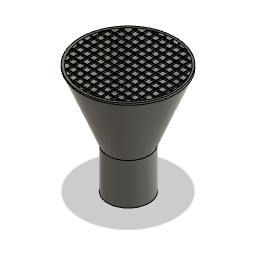
nose1 (Autodesk Fusion 360 design; units mm, degrees)
Autodesk Fusion 360 part; units mm, degrees
(part 1 of 3)
sketch "Sketch1" plane through (0, 0, 0) normal (0, 1, 0) x (1, 0, 0)
  circle A0 centre (0, 0) radius 15
  dimension "d1" = 30
  constraint coincident A0.centre origin
  measures "d1" diameter of A0
extrude "Extrude1" add sketch "Sketch1" along normal blind 30
ref_plane "WorkPlane1" through (0, 80, 0) normal (0, 1, 0) x (1, 0, 0)
sketch "Sketch2" plane through (0, 80, 0) normal (0, 1, 0) x (1, 0, 0)
  circle A0 centre (0, 0) radius 35
  constraint coincident A0.centre origin
loft "Loft1" add profiles "Sketch2" section 1 face at (0.9463, 30, 5.6032) section 2
shell "Shell1" thickness 2 removed faces 1 at (8.8451, 80, 11.8425)
sketch "Sketch3" plane through (0, 0, 0) normal (0, -1, 0) x (1, 0, 0)
  circle A0 centre (0, 0) radius 15
  circle A1 centre (0, 0) radius 13.5
  line L0 (-0.3, -13) -> (0.3, -13)
  line L1 (0.3, -13) -> (0.3, -16.7383)
  line L2 (0.3, -16.7383) -> (-0.3, -16.7383)
  line L3 (-0.3, -16.7383) -> (-0.3, -13)
  dimension "d6" = 27
  constraint coincident A0.centre A1.centre
  constraint horizontal L0
  constraint vertical L1
  constraint horizontal L2
  constraint vertical L3
  measures "d6" diameter of A1
extrude "Extrude2" cut sketch "Sketch3" against normal blind 37 contours A0 A1 L1 L3 | A0 L1 L2 L3 | A1 L0 L1 L3 | A1 L0 L1 L3 picked at (0.2333, -13.9978)
ref_plane "WorkPlane2" through (0, 81, 0) normal (0, 1, 0) x (0, 0, 1)
sketch "Sketch4" plane through (0, 81, 0) normal (0, 1, 0) x (1, 0, 0)
  circle A0 centre (0, 0) radius 35 construction
  line L0 (5, -30) -> (0.5, -30)
  line L1 (0.5, -30) -> (0.5, -25.5)
  line L2 (0.5, -25.5) -> (5, -25.5)
  line L3 (5, -25.5) -> (5, -30)
  line L4 (-4.5, -30) -> (-4.5, -25.5)
  line L5 (0, -25.5) -> (0, -30)
  line L6 (0, -30) -> (-4.5, -30)
  line L7 (-4.5, -25.5) -> (0, -25.5)
  line L8 (-14.5, -30) -> (-14.5, -25.5)
  line L9 (-9.5, -25.5) -> (-5, -25.5)
  line L10 (-10, -25.5) -> (-10, -30)
  line L11 (-14.5, -25.5) -> (-10, -25.5)
  line L12 (-5, -30) -> (-9.5, -30)
  line L13 (-5, -25.5) -> (-5, -30)
  line L14 (-9.5, -30) -> (-9.5, -25.5)
  line L15 (-10, -30) -> (-14.5, -30)
  line L16 (-24.5, -30) -> (-24.5, -25.5)
  line L17 (-19.5, -25.5) -> (-15, -25.5)
  line L18 (-20, -25.5) -> (-20, -30)
  line L19 (-24.5, -25.5) -> (-20, -25.5)
  line L20 (-15, -30) -> (-19.5, -30)
  line L21 (-15, -25.5) -> (-15, -30)
  line L22 (-19.5, -30) -> (-19.5, -25.5)
  line L23 (-20, -30) -> (-24.5, -30)
  line L24 (-34.5, -30) -> (-34.5, -25.5)
  line L25 (-29.5, -25.5) -> (-25, -25.5)
  line L26 (-30, -25.5) -> (-30, -30)
  line L27 (-34.5, -25.5) -> (-30, -25.5)
  line L28 (-25, -30) -> (-29.5, -30)
  line L29 (-25, -25.5) -> (-25, -30)
  line L30 (-29.5, -30) -> (-29.5, -25.5)
  line L31 (-30, -30) -> (-34.5, -30)
  line L32 (5.5, -30) -> (5.5, -25.5)
  line L33 (10.5, -25.5) -> (15, -25.5)
  line L34 (10, -25.5) -> (10, -30)
  line L35 (5.5, -25.5) -> (10, -25.5)
  line L36 (15, -30) -> (10.5, -30)
  line L37 (15, -25.5) -> (15, -30)
  line L38 (10.5, -30) -> (10.5, -25.5)
  line L39 (10, -30) -> (5.5, -30)
  line L40 (15.5, -30) -> (15.5, -25.5)
  line L41 (20.5, -25.5) -> (25, -25.5)
  line L42 (20, -25.5) -> (20, -30)
  line L43 (15.5, -25.5) -> (20, -25.5)
  line L44 (25, -30) -> (20.5, -30)
  line L45 (25, -25.5) -> (25, -30)
  line L46 (20.5, -30) -> (20.5, -25.5)
  line L47 (20, -30) -> (15.5, -30)
  line L48 (25.5, -30) -> (25.5, -25.5)
  line L49 (30.5, -25.5) -> (35, -25.5)
  line L50 (30, -25.5) -> (30, -30)
  line L51 (25.5, -25.5) -> (30, -25.5)
  line L52 (35, -30) -> (30.5, -30)
  line L53 (35, -25.5) -> (35, -30)
  line L54 (30.5, -30) -> (30.5, -25.5)
  line L55 (30, -30) -> (25.5, -30)
  line L56 (35, -25) -> (30.5, -25)
  line L57 (25, -20.5) -> (25, -25)
  line L58 (-14.5, -25) -> (-14.5, -20.5)
  line L59 (0.5, -25) -> (0.5, -20.5)
  line L60 (10.5, -20.5) -> (15, -20.5)
  line L61 (30.5, -25) -> (30.5, -20.5)
  line L62 (25.5, -20.5) -> (30, -20.5)
  line L63 (35, -20.5) -> (35, -25)
  line L64 (-5, -20.5) -> (-5, -25)
  line L65 (0, -25) -> (-4.5, -25)
  line L66 (5.5, -25) -> (5.5, -20.5)
  line L67 (15, -20.5) -> (15, -25)
  line L68 (30.5, -20.5) -> (35, -20.5)
  line L69 (20, -25) -> (15.5, -25)
  line L70 (20, -20.5) -> (20, -25)
  line L71 (5.5, -20.5) -> (10, -20.5)
  line L72 (10.5, -25) -> (10.5, -20.5)
  line L73 (10, -20.5) -> (10, -25)
  line L74 (0.5, -20.5) -> (5, -20.5)
  line L75 (-15, -20.5) -> (-15, -25)
  line L76 (-19.5, -20.5) -> (-15, -20.5)
  line L77 (-24.5, -25) -> (-24.5, -20.5)
  line L78 (-4.5, -25) -> (-4.5, -20.5)
  line L79 (-29.5, -25) -> (-29.5, -20.5)
  line L80 (-9.5, -20.5) -> (-5, -20.5)
  line L81 (-34.5, -25) -> (-34.5, -20.5)
  line L82 (-25, -20.5) -> (-25, -25)
  line L83 (-34.5, -20.5) -> (-30, -20.5)
  line L84 (-20, -25) -> (-24.5, -25)
  line L85 (20.5, -20.5) -> (25, -20.5)
  line L86 (5, -25) -> (0.5, -25)
  line L87 (-15, -25) -> (-19.5, -25)
  line L88 (-9.5, -25) -> (-9.5, -20.5)
  line L89 (30, -25) -> (25.5, -25)
  line L90 (25.5, -25) -> (25.5, -20.5)
  line L91 (30, -20.5) -> (30, -25)
  line L92 (-10, -20.5) -> (-10, -25)
  line L93 (10, -25) -> (5.5, -25)
  line L94 (-5, -25) -> (-9.5, -25)
  line L95 (15.5, -20.5) -> (20, -20.5)
  line L96 (-30, -25) -> (-34.5, -25)
  line L97 (15, -25) -> (10.5, -25)
  line L98 (-14.5, -20.5) -> (-10, -20.5)
  line L99 (-10, -25) -> (-14.5, -25)
  line L100 (20.5, -25) -> (20.5, -20.5)
  line L101 (25, -25) -> (20.5, -25)
  line L102 (15.5, -25) -> (15.5, -20.5)
  line L103 (5, -20.5) -> (5, -25)
  line L104 (-24.5, -20.5) -> (-20, -20.5)
  line L105 (-20, -20.5) -> (-20, -25)
  line L106 (-29.5, -20.5) -> (-25, -20.5)
  line L107 (-30, -20.5) -> (-30, -25)
  line L108 (-19.5, -25) -> (-19.5, -20.5)
  line L109 (0, -20.5) -> (0, -25)
  line L110 (-4.5, -20.5) -> (0, -20.5)
  line L111 (-25, -25) -> (-29.5, -25)
  line L112 (-5, -15) -> (-9.5, -15)
  line L113 (0, -10.5) -> (0, -15)
  line L114 (5, -15) -> (0.5, -15)
  line L115 (-9.5, -10.5) -> (-5, -10.5)
  line L116 (0.5, -15) -> (0.5, -10.5)
  line L117 (10, -15) -> (5.5, -15)
  line L118 (-4.5, -15) -> (-4.5, -10.5)
  line L119 (-10, -10.5) -> (-10, -15)
  line L120 (0, -15) -> (-4.5, -15)
  line L121 (-9.5, -15) -> (-9.5, -10.5)
  line L122 (15, -15) -> (10.5, -15)
  line L123 (15.5, -15) -> (15.5, -10.5)
  line L124 (30, -15.5) -> (30, -20)
  line L125 (-19.5, -20) -> (-19.5, -15.5)
  line L126 (20, -15) -> (15.5, -15)
  line L127 (10.5, -10.5) -> (15, -10.5)
  line L128 (-34.5, -15.5) -> (-30, -15.5)
  line L129 (-25, -15) -> (-29.5, -15)
  line L130 (35, -20) -> (30.5, -20)
  line L131 (25, -15) -> (20.5, -15)
  line L132 (25.5, -10.5) -> (30, -10.5)
  line L133 (25.5, -15) -> (25.5, -10.5)
  line L134 (30.5, -15) -> (30.5, -10.5)
  line L135 (35, -15) -> (30.5, -15)
  line L136 (15, -15.5) -> (15, -20)
  line L137 (-25, -20) -> (-29.5, -20)
  line L138 (15.5, -10.5) -> (20, -10.5)
  line L139 (-24.5, -10.5) -> (-20, -10.5)
  line L140 (-10, -15) -> (-14.5, -15)
  line L141 (-4.5, -20) -> (-4.5, -15.5)
  line L142 (0, -15.5) -> (0, -20)
  line L143 (-14.5, -10.5) -> (-10, -10.5)
  line L144 (-9.5, -15.5) -> (-5, -15.5)
  line L145 (-14.5, -15.5) -> (-10, -15.5)
  line L146 (-5, -15.5) -> (-5, -20)
  line L147 (5.5, -20) -> (5.5, -15.5)
  line L148 (5, -15.5) -> (5, -20)
  line L149 (5.5, -15.5) -> (10, -15.5)
  line L150 (0.5, -20) -> (0.5, -15.5)
  line L151 (-10, -20) -> (-14.5, -20)
  line L152 (-4.5, -10.5) -> (0, -10.5)
  line L153 (5.5, -15) -> (5.5, -10.5)
  line L154 (10, -10.5) -> (10, -15)
  line L155 (5, -10.5) -> (5, -15)
  line L156 (10.5, -15) -> (10.5, -10.5)
  line L157 (5.5, -10.5) -> (10, -10.5)
  line L158 (0.5, -10.5) -> (5, -10.5)
  line L159 (-10, -15.5) -> (-10, -20)
  line L160 (10, -15.5) -> (10, -20)
  line L161 (10.5, -20) -> (10.5, -15.5)
  line L162 (10, -20) -> (5.5, -20)
  line L163 (-19.5, -15.5) -> (-15, -15.5)
  line L164 (-34.5, -20) -> (-34.5, -15.5)
  line L165 (-15, -15.5) -> (-15, -20)
  line L166 (35, -10.5) -> (35, -15)
  line L167 (30.5, -20) -> (30.5, -15.5)
  line L168 (-25, -15.5) -> (-25, -20)
  line L169 (-20, -20) -> (-24.5, -20)
  line L170 (-15, -15) -> (-19.5, -15)
  line L171 (-29.5, -10.5) -> (-25, -10.5)
  line L172 (30.5, -10.5) -> (35, -10.5)
  line L173 (-29.5, -15.5) -> (-25, -15.5)
  line L174 (-30, -10.5) -> (-30, -15)
  line L175 (25, -10.5) -> (25, -15)
  line L176 (30, -15) -> (25.5, -15)
  line L177 (-14.5, -15) -> (-14.5, -10.5)
  line L178 (-20, -15) -> (-24.5, -15)
  line L179 (35, -15.5) -> (35, -20)
  line L180 (-19.5, -15) -> (-19.5, -10.5)
  line L181 (-34.5, -10.5) -> (-30, -10.5)
  line L182 (30, -20) -> (25.5, -20)
  line L183 (30, -10.5) -> (30, -15)
  line L184 (20.5, -10.5) -> (25, -10.5)
  line L185 (-24.5, -15) -> (-24.5, -10.5)
  line L186 (-15, -20) -> (-19.5, -20)
  line L187 (-29.5, -20) -> (-29.5, -15.5)
  line L188 (-20, -10.5) -> (-20, -15)
  line L189 (20.5, -15) -> (20.5, -10.5)
  line L190 (15, -10.5) -> (15, -15)
  line L191 (-24.5, -15.5) -> (-20, -15.5)
  line L192 (20, -10.5) -> (20, -15)
  line L193 (25.5, -20) -> (25.5, -15.5)
  line L194 (20.5, -15.5) -> (25, -15.5)
  line L195 (15.5, -15.5) -> (20, -15.5)
  line L196 (20, -20) -> (15.5, -20)
  line L197 (-25, -10.5) -> (-25, -15)
  line L198 (20, -15.5) -> (20, -20)
  line L199 (-15, -10.5) -> (-15, -15)
  line L200 (20.5, -20) -> (20.5, -15.5)
  line L201 (10.5, -15.5) -> (15, -15.5)
  line L202 (-20, -15.5) -> (-20, -20)
  line L203 (-30, -15) -> (-34.5, -15)
  line L204 (-30, -20) -> (-34.5, -20)
  line L205 (-34.5, -15) -> (-34.5, -10.5)
  line L206 (-30, -15.5) -> (-30, -20)
  line L207 (25, -15.5) -> (25, -20)
  line L208 (-29.5, -15) -> (-29.5, -10.5)
  line L209 (25, -20) -> (20.5, -20)
  line L210 (-24.5, -20) -> (-24.5, -15.5)
  line L211 (-14.5, -20) -> (-14.5, -15.5)
  line L212 (-19.5, -10.5) -> (-15, -10.5)
  line L213 (25.5, -15.5) -> (30, -15.5)
  line L214 (15.5, -20) -> (15.5, -15.5)
  line L215 (15, -20) -> (10.5, -20)
  line L216 (30.5, -15.5) -> (35, -15.5)
  line L217 (-5, -20) -> (-9.5, -20)
  line L218 (-5, -10.5) -> (-5, -15)
  line L219 (-4.5, -15.5) -> (0, -15.5)
  line L220 (0.5, -15.5) -> (5, -15.5)
  line L221 (-9.5, -20) -> (-9.5, -15.5)
  line L222 (0, -20) -> (-4.5, -20)
  line L223 (5, -20) -> (0.5, -20)
  line L224 (0.5, 4.5) -> (5, 4.5)
  line L225 (0.5, 9.5) -> (5, 9.5)
  line L226 (20.5, -5) -> (20.5, -0.5)
  line L227 (25, -5) -> (20.5, -5)
  line L228 (-10, -5) -> (-14.5, -5)
  line L229 (20.5, -10) -> (20.5, -5.5)
  line L230 (20, -10) -> (15.5, -10)
  line L231 (15, 4.5) -> (15, 0)
  line L232 (20, 5) -> (15.5, 5)
  line L233 (20, -5) -> (15.5, -5)
  line L234 (15.5, -5) -> (15.5, -0.5)
  line L235 (-14.5, -0.5) -> (-10, -0.5)
  line L236 (-10, 0) -> (-14.5, 0)
  line L237 (15.5, -5.5) -> (20, -5.5)
  line L238 (-10, 5) -> (-14.5, 5)
  line L239 (25, -10) -> (20.5, -10)
  line L240 (-10, -10) -> (-14.5, -10)
  line L241 (15, -5.5) -> (15, -10)
  line L242 (15.5, -0.5) -> (20, -0.5)
  line L243 (15, -0.5) -> (15, -5)
  line L244 (15.5, -10) -> (15.5, -5.5)
  line L245 (20.5, -0.5) -> (25, -0.5)
  line L246 (20.5, 5) -> (20.5, 9.5)
  line L247 (20, -0.5) -> (20, -5)
  line L248 (20, -5.5) -> (20, -10)
  line L249 (-14.5, -5.5) -> (-10, -5.5)
  line L250 (20, 0) -> (15.5, 0)
  line L251 (15.5, 5) -> (15.5, 9.5)
  line L252 (15.5, 9.5) -> (20, 9.5)
  line L253 (20.5, -5.5) -> (25, -5.5)
  line L254 (10, -5) -> (5.5, -5)
  line L255 (5.5, -5) -> (5.5, -0.5)
  line L256 (5.5, 0) -> (5.5, 4.5)
  line L257 (10, 5) -> (5.5, 5)
  line L258 (10, 4.5) -> (10, 0)
  line L259 (5.5, 5) -> (5.5, 9.5)
  line L260 (5.5, 9.5) -> (10, 9.5)
  line L261 (5.5, 4.5) -> (10, 4.5)
  line L262 (10, 9.5) -> (10, 5)
  line L263 (10.5, 5) -> (10.5, 9.5)
  line L264 (10, 0) -> (5.5, 0)
  line L265 (0, 4.5) -> (0, 0)
  line L266 (5, 9.5) -> (5, 5)
  line L267 (0, 9.5) -> (0, 5)
  line L268 (5, 5) -> (0.5, 5)
  line L269 (0.5, 0) -> (0.5, 4.5)
  line L270 (-10, -0.5) -> (-10, -5)
  line L271 (15, 9.5) -> (15, 5)
  line L272 (15.5, 4.5) -> (20, 4.5)
  line L273 (20, 4.5) -> (20, 0)
  line L274 (20, 9.5) -> (20, 5)
  line L275 (-4.5, 9.5) -> (0, 9.5)
  line L276 (0, 5) -> (-4.5, 5)
  line L277 (-4.5, -0.5) -> (0, -0.5)
  line L278 (15.5, 0) -> (15.5, 4.5)
  line L279 (-9.5, -0.5) -> (-5, -0.5)
  line L280 (0, 0) -> (-4.5, 0)
  line L281 (0, -10) -> (-4.5, -10)
  line L282 (-5, -5) -> (-9.5, -5)
  line L283 (-4.5, -5.5) -> (0, -5.5)
  line L284 (-4.5, 4.5) -> (0, 4.5)
  line L285 (20.5, 0) -> (20.5, 4.5)
  line L286 (-10, -5.5) -> (-10, -10)
  line L287 (0, -5) -> (-4.5, -5)
  line L288 (-5, -0.5) -> (-5, -5)
  line L289 (-5, -10) -> (-9.5, -10)
  line L290 (-9.5, -10) -> (-9.5, -5.5)
  line L291 (-5, -5.5) -> (-5, -10)
  line L292 (-5, 5) -> (-9.5, 5)
  line L293 (-9.5, -5.5) -> (-5, -5.5)
  line L294 (-9.5, 9.5) -> (-5, 9.5)
  line L295 (-9.5, 4.5) -> (-5, 4.5)
  line L296 (-5, 0) -> (-9.5, 0)
  line L297 (-4.5, 5) -> (-4.5, 9.5)
  line L298 (-9.5, -5) -> (-9.5, -0.5)
  line L299 (-5, 9.5) -> (-5, 5)
  line L300 (-4.5, -10) -> (-4.5, -5.5)
  line L301 (-4.5, -5) -> (-4.5, -0.5)
  line L302 (-10, 4.5) -> (-10, 0)
  line L303 (-9.5, 5) -> (-9.5, 9.5)
  line L304 (-10, 9.5) -> (-10, 5)
  line L305 (-4.5, 0) -> (-4.5, 4.5)
  line L306 (-5, 4.5) -> (-5, 0)
  line L307 (-9.5, 0) -> (-9.5, 4.5)
  line L308 (10, -0.5) -> (10, -5)
  line L309 (10.5, -5) -> (10.5, -0.5)
  line L310 (10, -5.5) -> (10, -10)
  line L311 (5.5, -10) -> (5.5, -5.5)
  line L312 (10.5, -10) -> (10.5, -5.5)
  line L313 (5.5, -0.5) -> (10, -0.5)
  line L314 (10, -10) -> (5.5, -10)
  line L315 (5.5, -5.5) -> (10, -5.5)
  line L316 (-20, 5) -> (-24.5, 5)
  line L317 (35, 9.5) -> (35, 5)
  line L318 (15, 5) -> (10.5, 5)
  line L319 (30.5, 5) -> (30.5, 9.5)
  line L320 (35, 4.5) -> (35, 0)
  line L321 (-14.5, 5) -> (-14.5, 9.5)
  line L322 (35, 5) -> (30.5, 5)
  line L323 (10.5, -5.5) -> (15, -5.5)
  line L324 (-29.5, -0.5) -> (-25, -0.5)
  line L325 (25, 5) -> (20.5, 5)
  line L326 (-19.5, -5.5) -> (-15, -5.5)
  line L327 (-30, -5.5) -> (-30, -10)
  line L328 (30.5, 9.5) -> (35, 9.5)
  line L329 (-14.5, 4.5) -> (-10, 4.5)
  line L330 (25, 9.5) -> (25, 5)
  line L331 (30, 0) -> (25.5, 0)
  line L332 (-24.5, 9.5) -> (-20, 9.5)
  line L333 (-24.5, -5.5) -> (-20, -5.5)
  line L334 (15, 0) -> (10.5, 0)
  line L335 (-20, 9.5) -> (-20, 5)
  line L336 (-24.5, -0.5) -> (-20, -0.5)
  line L337 (25.5, 5) -> (25.5, 9.5)
  line L338 (30, 5) -> (25.5, 5)
  line L339 (25, 4.5) -> (25, 0)
  line L340 (35, 0) -> (30.5, 0)
  line L341 (25.5, 9.5) -> (30, 9.5)
  line L342 (-20, 0) -> (-24.5, 0)
  line L343 (-30, -5) -> (-34.5, -5)
  line L344 (-19.5, 9.5) -> (-15, 9.5)
  line L345 (-14.5, 0) -> (-14.5, 4.5)
  line L346 (-19.5, 5) -> (-19.5, 9.5)
  line L347 (10.5, 9.5) -> (15, 9.5)
  line L348 (-19.5, -5) -> (-19.5, -0.5)
  line L349 (-19.5, 4.5) -> (-15, 4.5)
  line L350 (10.5, 4.5) -> (15, 4.5)
  line L351 (25.5, 0) -> (25.5, 4.5)
  line L352 (15, -5) -> (10.5, -5)
  line L353 (30, 9.5) -> (30, 5)
  line L354 (-14.5, 9.5) -> (-10, 9.5)
  line L355 (-24.5, 4.5) -> (-20, 4.5)
  line L356 (15, -10) -> (10.5, -10)
  line L357 (10.5, -0.5) -> (15, -0.5)
  line L358 (10.5, 0) -> (10.5, 4.5)
  line L359 (0, -5.5) -> (0, -10)
  line L360 (5, -0.5) -> (5, -5)
  line L361 (-34.5, -5.5) -> (-30, -5.5)
  line L362 (30.5, -10) -> (30.5, -5.5)
  line L363 (-25, 4.5) -> (-25, 0)
  line L364 (-34.5, 0) -> (-34.5, 4.5)
  line L365 (-25, 0) -> (-29.5, 0)
  line L366 (-29.5, -5) -> (-29.5, -0.5)
  line L367 (30, -0.5) -> (30, -5)
  line L368 (25, -5.5) -> (25, -10)
  line L369 (30.5, -5.5) -> (35, -5.5)
  line L370 (-29.5, 9.5) -> (-25, 9.5)
  line L371 (30, -5) -> (25.5, -5)
  line L372 (25.5, -0.5) -> (30, -0.5)
  line L373 (-34.5, -10) -> (-34.5, -5.5)
  line L374 (-30, 4.5) -> (-30, 0)
  line L375 (-29.5, -10) -> (-29.5, -5.5)
  line L376 (-25, -10) -> (-29.5, -10)
  line L377 (-29.5, 5) -> (-29.5, 9.5)
  line L378 (-25, 9.5) -> (-25, 5)
  line L379 (-29.5, -5.5) -> (-25, -5.5)
  line L380 (-34.5, -5) -> (-34.5, -0.5)
  line L381 (-34.5, 4.5) -> (-30, 4.5)
  line L382 (-34.5, 5) -> (-34.5, 9.5)
  line L383 (-29.5, 4.5) -> (-25, 4.5)
  line L384 (-30, -0.5) -> (-30, -5)
  line L385 (-24.5, -10) -> (-24.5, -5.5)
  line L386 (30, -5.5) -> (30, -10)
  line L387 (-25, -5) -> (-29.5, -5)
  line L388 (-34.5, -0.5) -> (-30, -0.5)
  line L389 (-19.5, -10) -> (-19.5, -5.5)
  line L390 (-25, 5) -> (-29.5, 5)
  line L391 (35, -10) -> (30.5, -10)
  line L392 (-15, 5) -> (-19.5, 5)
  line L393 (-30, 9.5) -> (-30, 5)
  line L394 (-20, -0.5) -> (-20, -5)
  line L395 (-30, 0) -> (-34.5, 0)
  line L396 (-14.5, -5) -> (-14.5, -0.5)
  line L397 (-24.5, -5) -> (-24.5, -0.5)
  line L398 (30.5, 4.5) -> (35, 4.5)
  line L399 (-25, -5.5) -> (-25, -10)
  line L400 (30, 4.5) -> (30, 0)
  line L401 (-19.5, -0.5) -> (-15, -0.5)
  line L402 (-20, -5.5) -> (-20, -10)
  line L403 (30, -10) -> (25.5, -10)
  line L404 (-15, 0) -> (-19.5, 0)
  line L405 (25.5, 4.5) -> (30, 4.5)
  line L406 (30.5, 0) -> (30.5, 4.5)
  line L407 (25, -0.5) -> (25, -5)
  line L408 (-19.5, 0) -> (-19.5, 4.5)
  line L409 (-15, 9.5) -> (-15, 5)
  line L410 (35, -5.5) -> (35, -10)
  line L411 (-29.5, 0) -> (-29.5, 4.5)
  line L412 (-24.5, 5) -> (-24.5, 9.5)
  line L413 (-15, -5.5) -> (-15, -10)
  line L414 (25.5, -5) -> (25.5, -0.5)
  line L415 (30.5, -0.5) -> (35, -0.5)
  line L416 (-15, -0.5) -> (-15, -5)
  line L417 (-34.5, 9.5) -> (-30, 9.5)
  line L418 (-20, 4.5) -> (-20, 0)
  line L419 (25, 0) -> (20.5, 0)
  line L420 (-24.5, 0) -> (-24.5, 4.5)
  line L421 (-20, -10) -> (-24.5, -10)
  line L422 (-15, 4.5) -> (-15, 0)
  line L423 (25.5, -10) -> (25.5, -5.5)
  line L424 (30.5, -5) -> (30.5, -0.5)
  line L425 (-25, -0.5) -> (-25, -5)
  line L426 (-15, -5) -> (-19.5, -5)
  line L427 (35, -5) -> (30.5, -5)
  line L428 (-30, -10) -> (-34.5, -10)
  line L429 (35, -0.5) -> (35, -5)
  line L430 (-14.5, -10) -> (-14.5, -5.5)
  line L431 (20.5, 4.5) -> (25, 4.5)
  line L432 (-20, -5) -> (-24.5, -5)
  line L433 (-30, 5) -> (-34.5, 5)
  line L434 (-15, -10) -> (-19.5, -10)
  line L435 (25.5, -5.5) -> (30, -5.5)
  line L436 (20.5, 9.5) -> (25, 9.5)
  line L437 (5, -5) -> (0.5, -5)
  line L438 (5, -5.5) -> (5, -10)
  line L439 (5, -10) -> (0.5, -10)
  line L440 (0.5, -10) -> (0.5, -5.5)
  line L441 (0.5, -5.5) -> (5, -5.5)
  line L442 (0.5, -0.5) -> (5, -0.5)
  line L443 (5, 4.5) -> (5, 0)
  line L444 (0.5, 5) -> (0.5, 9.5)
  line L445 (5, 0) -> (0.5, 0)
  line L446 (0, -0.5) -> (0, -5)
  line L447 (0.5, -5) -> (0.5, -0.5)
  line L448 (0.5, -15.5) -> (5, -15.5)
  line L449 (0.5, -10.5) -> (5, -10.5)
  line L450 (20.5, -25) -> (20.5, -20.5)
  line L451 (25, -25) -> (20.5, -25)
  line L452 (-10, -25) -> (-14.5, -25)
  line L453 (20.5, -30) -> (20.5, -25.5)
  line L454 (20, -30) -> (15.5, -30)
  line L455 (15, -15.5) -> (15, -20)
  line L456 (20, -15) -> (15.5, -15)
  line L457 (20, -25) -> (15.5, -25)
  line L458 (15.5, -25) -> (15.5, -20.5)
  line L459 (-14.5, -20.5) -> (-10, -20.5)
  line L460 (-10, -20) -> (-14.5, -20)
  line L461 (15.5, -25.5) -> (20, -25.5)
  line L462 (-10, -15) -> (-14.5, -15)
  line L463 (25, -30) -> (20.5, -30)
  line L464 (-10, -30) -> (-14.5, -30)
  line L465 (15, -25.5) -> (15, -30)
  line L466 (15.5, -20.5) -> (20, -20.5)
  line L467 (15, -20.5) -> (15, -25)
  line L468 (15.5, -30) -> (15.5, -25.5)
  line L469 (20.5, -20.5) -> (25, -20.5)
  line L470 (20.5, -15) -> (20.5, -10.5)
  line L471 (20, -20.5) -> (20, -25)
  line L472 (20, -25.5) -> (20, -30)
  line L473 (-14.5, -25.5) -> (-10, -25.5)
  line L474 (20, -20) -> (15.5, -20)
  line L475 (15.5, -15) -> (15.5, -10.5)
  line L476 (15.5, -10.5) -> (20, -10.5)
  line L477 (20.5, -25.5) -> (25, -25.5)
  line L478 (10, -25) -> (5.5, -25)
  line L479 (5.5, -25) -> (5.5, -20.5)
  line L480 (5.5, -20) -> (5.5, -15.5)
  line L481 (10, -15) -> (5.5, -15)
  line L482 (10, -15.5) -> (10, -20)
  line L483 (5.5, -15) -> (5.5, -10.5)
  line L484 (5.5, -10.5) -> (10, -10.5)
  line L485 (5.5, -15.5) -> (10, -15.5)
  line L486 (10, -10.5) -> (10, -15)
  line L487 (10.5, -15) -> (10.5, -10.5)
  line L488 (10, -20) -> (5.5, -20)
  line L489 (0, -15.5) -> (0, -20)
  line L490 (5, -10.5) -> (5, -15)
  line L491 (0, -10.5) -> (0, -15)
  line L492 (5, -15) -> (0.5, -15)
  line L493 (0.5, -20) -> (0.5, -15.5)
  line L494 (-10, -20.5) -> (-10, -25)
  line L495 (15, -10.5) -> (15, -15)
  line L496 (15.5, -15.5) -> (20, -15.5)
  line L497 (20, -15.5) -> (20, -20)
  line L498 (20, -10.5) -> (20, -15)
  line L499 (-4.5, -10.5) -> (0, -10.5)
  line L500 (0, -15) -> (-4.5, -15)
  line L501 (-4.5, -20.5) -> (0, -20.5)
  line L502 (15.5, -20) -> (15.5, -15.5)
  line L503 (-9.5, -20.5) -> (-5, -20.5)
  line L504 (0, -20) -> (-4.5, -20)
  line L505 (0, -30) -> (-4.5, -30)
  line L506 (-5, -25) -> (-9.5, -25)
  line L507 (-4.5, -25.5) -> (0, -25.5)
  line L508 (-4.5, -15.5) -> (0, -15.5)
  line L509 (20.5, -20) -> (20.5, -15.5)
  line L510 (-10, -25.5) -> (-10, -30)
  line L511 (0, -25) -> (-4.5, -25)
  line L512 (-5, -20.5) -> (-5, -25)
  line L513 (-5, -30) -> (-9.5, -30)
  line L514 (-9.5, -30) -> (-9.5, -25.5)
  line L515 (-5, -25.5) -> (-5, -30)
  line L516 (-5, -15) -> (-9.5, -15)
  line L517 (-9.5, -25.5) -> (-5, -25.5)
  line L518 (-9.5, -10.5) -> (-5, -10.5)
  line L519 (-9.5, -15.5) -> (-5, -15.5)
  line L520 (-5, -20) -> (-9.5, -20)
  line L521 (-4.5, -15) -> (-4.5, -10.5)
  line L522 (-9.5, -25) -> (-9.5, -20.5)
  line L523 (-5, -10.5) -> (-5, -15)
  line L524 (-4.5, -30) -> (-4.5, -25.5)
  line L525 (-4.5, -25) -> (-4.5, -20.5)
  line L526 (-10, -15.5) -> (-10, -20)
  line L527 (-9.5, -15) -> (-9.5, -10.5)
  line L528 (-10, -10.5) -> (-10, -15)
  line L529 (-4.5, -20) -> (-4.5, -15.5)
  line L530 (-5, -15.5) -> (-5, -20)
  line L531 (-9.5, -20) -> (-9.5, -15.5)
  line L532 (10, -20.5) -> (10, -25)
  line L533 (10.5, -25) -> (10.5, -20.5)
  line L534 (10, -25.5) -> (10, -30)
  line L535 (5.5, -30) -> (5.5, -25.5)
  line L536 (10.5, -30) -> (10.5, -25.5)
  line L537 (5.5, -20.5) -> (10, -20.5)
  line L538 (10, -30) -> (5.5, -30)
  line L539 (5.5, -25.5) -> (10, -25.5)
  line L540 (-20, -15) -> (-24.5, -15)
  line L541 (35, -10.5) -> (35, -15)
  line L542 (15, -15) -> (10.5, -15)
  line L543 (30.5, -15) -> (30.5, -10.5)
  line L544 (35, -15.5) -> (35, -20)
  line L545 (-14.5, -15) -> (-14.5, -10.5)
  line L546 (35, -15) -> (30.5, -15)
  line L547 (10.5, -25.5) -> (15, -25.5)
  line L548 (-29.5, -20.5) -> (-25, -20.5)
  line L549 (25, -15) -> (20.5, -15)
  line L550 (-19.5, -25.5) -> (-15, -25.5)
  line L551 (-30, -25.5) -> (-30, -30)
  line L552 (30.5, -10.5) -> (35, -10.5)
  line L553 (-14.5, -15.5) -> (-10, -15.5)
  line L554 (25, -10.5) -> (25, -15)
  line L555 (30, -20) -> (25.5, -20)
  line L556 (-24.5, -10.5) -> (-20, -10.5)
  line L557 (-24.5, -25.5) -> (-20, -25.5)
  line L558 (15, -20) -> (10.5, -20)
  line L559 (-20, -10.5) -> (-20, -15)
  line L560 (-24.5, -20.5) -> (-20, -20.5)
  line L561 (25.5, -15) -> (25.5, -10.5)
  line L562 (30, -15) -> (25.5, -15)
  line L563 (25, -15.5) -> (25, -20)
  line L564 (35, -20) -> (30.5, -20)
  line L565 (25.5, -10.5) -> (30, -10.5)
  line L566 (-20, -20) -> (-24.5, -20)
  line L567 (-30, -25) -> (-34.5, -25)
  line L568 (-19.5, -10.5) -> (-15, -10.5)
  line L569 (-14.5, -20) -> (-14.5, -15.5)
  line L570 (-19.5, -15) -> (-19.5, -10.5)
  line L571 (10.5, -10.5) -> (15, -10.5)
  line L572 (-19.5, -25) -> (-19.5, -20.5)
  line L573 (-19.5, -15.5) -> (-15, -15.5)
  line L574 (10.5, -15.5) -> (15, -15.5)
  line L575 (25.5, -20) -> (25.5, -15.5)
  line L576 (15, -25) -> (10.5, -25)
  line L577 (30, -10.5) -> (30, -15)
  line L578 (-14.5, -10.5) -> (-10, -10.5)
  line L579 (-24.5, -15.5) -> (-20, -15.5)
  line L580 (15, -30) -> (10.5, -30)
  line L581 (10.5, -20.5) -> (15, -20.5)
  line L582 (10.5, -20) -> (10.5, -15.5)
  line L583 (0, -25.5) -> (0, -30)
  line L584 (5, -20.5) -> (5, -25)
  line L585 (-34.5, -25.5) -> (-30, -25.5)
  line L586 (30.5, -30) -> (30.5, -25.5)
  line L587 (-25, -15.5) -> (-25, -20)
  line L588 (-34.5, -20) -> (-34.5, -15.5)
  line L589 (-25, -20) -> (-29.5, -20)
  line L590 (-29.5, -25) -> (-29.5, -20.5)
  line L591 (30, -20.5) -> (30, -25)
  line L592 (25, -25.5) -> (25, -30)
  line L593 (30.5, -25.5) -> (35, -25.5)
  line L594 (-29.5, -10.5) -> (-25, -10.5)
  line L595 (30, -25) -> (25.5, -25)
  line L596 (25.5, -20.5) -> (30, -20.5)
  line L597 (-34.5, -30) -> (-34.5, -25.5)
  line L598 (-30, -15.5) -> (-30, -20)
  line L599 (-29.5, -30) -> (-29.5, -25.5)
  line L600 (-25, -30) -> (-29.5, -30)
  line L601 (-29.5, -15) -> (-29.5, -10.5)
  line L602 (-25, -10.5) -> (-25, -15)
  line L603 (-29.5, -25.5) -> (-25, -25.5)
  line L604 (-34.5, -25) -> (-34.5, -20.5)
  line L605 (-34.5, -15.5) -> (-30, -15.5)
  line L606 (-34.5, -15) -> (-34.5, -10.5)
  line L607 (-29.5, -15.5) -> (-25, -15.5)
  line L608 (-30, -20.5) -> (-30, -25)
  line L609 (-24.5, -30) -> (-24.5, -25.5)
  line L610 (30, -25.5) -> (30, -30)
  line L611 (-25, -25) -> (-29.5, -25)
  line L612 (-34.5, -20.5) -> (-30, -20.5)
  line L613 (-19.5, -30) -> (-19.5, -25.5)
  line L614 (-25, -15) -> (-29.5, -15)
  line L615 (35, -30) -> (30.5, -30)
  line L616 (-15, -15) -> (-19.5, -15)
  line L617 (-30, -10.5) -> (-30, -15)
  line L618 (-20, -20.5) -> (-20, -25)
  line L619 (-30, -20) -> (-34.5, -20)
  line L620 (-14.5, -25) -> (-14.5, -20.5)
  line L621 (-24.5, -25) -> (-24.5, -20.5)
  line L622 (30.5, -15.5) -> (35, -15.5)
  line L623 (-25, -25.5) -> (-25, -30)
  line L624 (30, -15.5) -> (30, -20)
  line L625 (-19.5, -20.5) -> (-15, -20.5)
  line L626 (-20, -25.5) -> (-20, -30)
  line L627 (30, -30) -> (25.5, -30)
  line L628 (-15, -20) -> (-19.5, -20)
  line L629 (25.5, -15.5) -> (30, -15.5)
  line L630 (30.5, -20) -> (30.5, -15.5)
  line L631 (25, -20.5) -> (25, -25)
  line L632 (-19.5, -20) -> (-19.5, -15.5)
  line L633 (-15, -10.5) -> (-15, -15)
  line L634 (35, -25.5) -> (35, -30)
  line L635 (-29.5, -20) -> (-29.5, -15.5)
  line L636 (-24.5, -15) -> (-24.5, -10.5)
  line L637 (-15, -25.5) -> (-15, -30)
  line L638 (25.5, -25) -> (25.5, -20.5)
  line L639 (30.5, -20.5) -> (35, -20.5)
  line L640 (-15, -20.5) -> (-15, -25)
  line L641 (-34.5, -10.5) -> (-30, -10.5)
  line L642 (-20, -15.5) -> (-20, -20)
  line L643 (25, -20) -> (20.5, -20)
  line L644 (-24.5, -20) -> (-24.5, -15.5)
  line L645 (-20, -30) -> (-24.5, -30)
  line L646 (-15, -15.5) -> (-15, -20)
  line L647 (25.5, -30) -> (25.5, -25.5)
  line L648 (30.5, -25) -> (30.5, -20.5)
  line L649 (-25, -20.5) -> (-25, -25)
  line L650 (-15, -25) -> (-19.5, -25)
  line L651 (35, -25) -> (30.5, -25)
  line L652 (-30, -30) -> (-34.5, -30)
  line L653 (35, -20.5) -> (35, -25)
  line L654 (-14.5, -30) -> (-14.5, -25.5)
  line L655 (20.5, -15.5) -> (25, -15.5)
  line L656 (-20, -25) -> (-24.5, -25)
  line L657 (-30, -15) -> (-34.5, -15)
  line L658 (-15, -30) -> (-19.5, -30)
  line L659 (25.5, -25.5) -> (30, -25.5)
  line L660 (20.5, -10.5) -> (25, -10.5)
  line L661 (5, -25) -> (0.5, -25)
  line L662 (5, -25.5) -> (5, -30)
  line L663 (5, -30) -> (0.5, -30)
  line L664 (0.5, -30) -> (0.5, -25.5)
  line L665 (0.5, -25.5) -> (5, -25.5)
  line L666 (0.5, -20.5) -> (5, -20.5)
  line L667 (5, -15.5) -> (5, -20)
  line L668 (0.5, -15) -> (0.5, -10.5)
  line L669 (5, -20) -> (0.5, -20)
  line L670 (0, -20.5) -> (0, -25)
  line L671 (0.5, -25) -> (0.5, -20.5)
  line L672 (0.5, 24.5) -> (5, 24.5)
  line L673 (0.5, 29.5) -> (5, 29.5)
  line L674 (20.5, 15) -> (20.5, 19.5)
  line L675 (25, 15) -> (20.5, 15)
  line L676 (-10, 15) -> (-14.5, 15)
  line L677 (20.5, 10) -> (20.5, 14.5)
  line L678 (20, 10) -> (15.5, 10)
  line L679 (15, 24.5) -> (15, 20)
  line L680 (20, 25) -> (15.5, 25)
  line L681 (20, 15) -> (15.5, 15)
  line L682 (15.5, 15) -> (15.5, 19.5)
  line L683 (-14.5, 19.5) -> (-10, 19.5)
  line L684 (-10, 20) -> (-14.5, 20)
  line L685 (15.5, 14.5) -> (20, 14.5)
  line L686 (-10, 25) -> (-14.5, 25)
  line L687 (25, 10) -> (20.5, 10)
  line L688 (-10, 10) -> (-14.5, 10)
  line L689 (15, 14.5) -> (15, 10)
  line L690 (15.5, 19.5) -> (20, 19.5)
  line L691 (15, 19.5) -> (15, 15)
  line L692 (15.5, 10) -> (15.5, 14.5)
  line L693 (20.5, 19.5) -> (25, 19.5)
  line L694 (20.5, 25) -> (20.5, 29.5)
  line L695 (20, 19.5) -> (20, 15)
  line L696 (20, 14.5) -> (20, 10)
  line L697 (-14.5, 14.5) -> (-10, 14.5)
  line L698 (20, 20) -> (15.5, 20)
  line L699 (15.5, 25) -> (15.5, 29.5)
  line L700 (15.5, 29.5) -> (20, 29.5)
  line L701 (20.5, 14.5) -> (25, 14.5)
  line L702 (10, 15) -> (5.5, 15)
  line L703 (5.5, 15) -> (5.5, 19.5)
  line L704 (5.5, 20) -> (5.5, 24.5)
  line L705 (10, 25) -> (5.5, 25)
  line L706 (10, 24.5) -> (10, 20)
  line L707 (5.5, 25) -> (5.5, 29.5)
  line L708 (5.5, 29.5) -> (10, 29.5)
  line L709 (5.5, 24.5) -> (10, 24.5)
  line L710 (10, 29.5) -> (10, 25)
  line L711 (10.5, 25) -> (10.5, 29.5)
  line L712 (10, 20) -> (5.5, 20)
  line L713 (0, 24.5) -> (0, 20)
  line L714 (5, 29.5) -> (5, 25)
  line L715 (0, 29.5) -> (0, 25)
  line L716 (5, 25) -> (0.5, 25)
  line L717 (0.5, 20) -> (0.5, 24.5)
  line L718 (-10, 19.5) -> (-10, 15)
  line L719 (15, 29.5) -> (15, 25)
  line L720 (15.5, 24.5) -> (20, 24.5)
  line L721 (20, 24.5) -> (20, 20)
  line L722 (20, 29.5) -> (20, 25)
  line L723 (-4.5, 29.5) -> (0, 29.5)
  line L724 (0, 25) -> (-4.5, 25)
  line L725 (-4.5, 19.5) -> (0, 19.5)
  line L726 (15.5, 20) -> (15.5, 24.5)
  line L727 (-9.5, 19.5) -> (-5, 19.5)
  line L728 (0, 20) -> (-4.5, 20)
  line L729 (0, 10) -> (-4.5, 10)
  line L730 (-5, 15) -> (-9.5, 15)
  line L731 (-4.5, 14.5) -> (0, 14.5)
  line L732 (-4.5, 24.5) -> (0, 24.5)
  line L733 (20.5, 20) -> (20.5, 24.5)
  line L734 (-10, 14.5) -> (-10, 10)
  line L735 (0, 15) -> (-4.5, 15)
  line L736 (-5, 19.5) -> (-5, 15)
  line L737 (-5, 10) -> (-9.5, 10)
  line L738 (-9.5, 10) -> (-9.5, 14.5)
  line L739 (-5, 14.5) -> (-5, 10)
  line L740 (-5, 25) -> (-9.5, 25)
  line L741 (-9.5, 14.5) -> (-5, 14.5)
  line L742 (-9.5, 29.5) -> (-5, 29.5)
  line L743 (-9.5, 24.5) -> (-5, 24.5)
  line L744 (-5, 20) -> (-9.5, 20)
  line L745 (-4.5, 25) -> (-4.5, 29.5)
  line L746 (-9.5, 15) -> (-9.5, 19.5)
  line L747 (-5, 29.5) -> (-5, 25)
  line L748 (-4.5, 10) -> (-4.5, 14.5)
  line L749 (-4.5, 15) -> (-4.5, 19.5)
  line L750 (-10, 24.5) -> (-10, 20)
  line L751 (-9.5, 25) -> (-9.5, 29.5)
  line L752 (-10, 29.5) -> (-10, 25)
  line L753 (-4.5, 20) -> (-4.5, 24.5)
  line L754 (-5, 24.5) -> (-5, 20)
  line L755 (-9.5, 20) -> (-9.5, 24.5)
  line L756 (10, 19.5) -> (10, 15)
  line L757 (10.5, 15) -> (10.5, 19.5)
  line L758 (10, 14.5) -> (10, 10)
  line L759 (5.5, 10) -> (5.5, 14.5)
  line L760 (10.5, 10) -> (10.5, 14.5)
  line L761 (5.5, 19.5) -> (10, 19.5)
  line L762 (10, 10) -> (5.5, 10)
  line L763 (5.5, 14.5) -> (10, 14.5)
  line L764 (-20, 25) -> (-24.5, 25)
  line L765 (35, 29.5) -> (35, 25)
  line L766 (15, 25) -> (10.5, 25)
  line L767 (30.5, 25) -> (30.5, 29.5)
  line L768 (35, 24.5) -> (35, 20)
  line L769 (-14.5, 25) -> (-14.5, 29.5)
  line L770 (35, 25) -> (30.5, 25)
  line L771 (10.5, 14.5) -> (15, 14.5)
  line L772 (-29.5, 19.5) -> (-25, 19.5)
  line L773 (25, 25) -> (20.5, 25)
  line L774 (-19.5, 14.5) -> (-15, 14.5)
  line L775 (-30, 14.5) -> (-30, 10)
  line L776 (30.5, 29.5) -> (35, 29.5)
  line L777 (-14.5, 24.5) -> (-10, 24.5)
  line L778 (25, 29.5) -> (25, 25)
  line L779 (30, 20) -> (25.5, 20)
  line L780 (-24.5, 29.5) -> (-20, 29.5)
  line L781 (-24.5, 14.5) -> (-20, 14.5)
  line L782 (15, 20) -> (10.5, 20)
  line L783 (-20, 29.5) -> (-20, 25)
  line L784 (-24.5, 19.5) -> (-20, 19.5)
  line L785 (25.5, 25) -> (25.5, 29.5)
  line L786 (30, 25) -> (25.5, 25)
  line L787 (25, 24.5) -> (25, 20)
  line L788 (35, 20) -> (30.5, 20)
  line L789 (25.5, 29.5) -> (30, 29.5)
  line L790 (-20, 20) -> (-24.5, 20)
  line L791 (-30, 15) -> (-34.5, 15)
  line L792 (-19.5, 29.5) -> (-15, 29.5)
  line L793 (-14.5, 20) -> (-14.5, 24.5)
  line L794 (-19.5, 25) -> (-19.5, 29.5)
  line L795 (10.5, 29.5) -> (15, 29.5)
  line L796 (-19.5, 15) -> (-19.5, 19.5)
  line L797 (-19.5, 24.5) -> (-15, 24.5)
  line L798 (10.5, 24.5) -> (15, 24.5)
  line L799 (25.5, 20) -> (25.5, 24.5)
  line L800 (15, 15) -> (10.5, 15)
  line L801 (30, 29.5) -> (30, 25)
  line L802 (-14.5, 29.5) -> (-10, 29.5)
  line L803 (-24.5, 24.5) -> (-20, 24.5)
  line L804 (15, 10) -> (10.5, 10)
  line L805 (10.5, 19.5) -> (15, 19.5)
  line L806 (10.5, 20) -> (10.5, 24.5)
  line L807 (0, 14.5) -> (0, 10)
  line L808 (5, 19.5) -> (5, 15)
  line L809 (-34.5, 14.5) -> (-30, 14.5)
  line L810 (30.5, 10) -> (30.5, 14.5)
  line L811 (-25, 24.5) -> (-25, 20)
  line L812 (-34.5, 20) -> (-34.5, 24.5)
  line L813 (-25, 20) -> (-29.5, 20)
  line L814 (-29.5, 15) -> (-29.5, 19.5)
  line L815 (30, 19.5) -> (30, 15)
  line L816 (25, 14.5) -> (25, 10)
  line L817 (30.5, 14.5) -> (35, 14.5)
  line L818 (-29.5, 29.5) -> (-25, 29.5)
  line L819 (30, 15) -> (25.5, 15)
  line L820 (25.5, 19.5) -> (30, 19.5)
  line L821 (-34.5, 10) -> (-34.5, 14.5)
  line L822 (-30, 24.5) -> (-30, 20)
  line L823 (-29.5, 10) -> (-29.5, 14.5)
  line L824 (-25, 10) -> (-29.5, 10)
  line L825 (-29.5, 25) -> (-29.5, 29.5)
  line L826 (-25, 29.5) -> (-25, 25)
  line L827 (-29.5, 14.5) -> (-25, 14.5)
  line L828 (-34.5, 15) -> (-34.5, 19.5)
  line L829 (-34.5, 24.5) -> (-30, 24.5)
  line L830 (-34.5, 25) -> (-34.5, 29.5)
  line L831 (-29.5, 24.5) -> (-25, 24.5)
  line L832 (-30, 19.5) -> (-30, 15)
  line L833 (-24.5, 10) -> (-24.5, 14.5)
  line L834 (30, 14.5) -> (30, 10)
  line L835 (-25, 15) -> (-29.5, 15)
  line L836 (-34.5, 19.5) -> (-30, 19.5)
  line L837 (-19.5, 10) -> (-19.5, 14.5)
  line L838 (-25, 25) -> (-29.5, 25)
  line L839 (35, 10) -> (30.5, 10)
  line L840 (-15, 25) -> (-19.5, 25)
  line L841 (-30, 29.5) -> (-30, 25)
  line L842 (-20, 19.5) -> (-20, 15)
  line L843 (-30, 20) -> (-34.5, 20)
  line L844 (-14.5, 15) -> (-14.5, 19.5)
  line L845 (-24.5, 15) -> (-24.5, 19.5)
  line L846 (30.5, 24.5) -> (35, 24.5)
  line L847 (-25, 14.5) -> (-25, 10)
  line L848 (30, 24.5) -> (30, 20)
  line L849 (-19.5, 19.5) -> (-15, 19.5)
  line L850 (-20, 14.5) -> (-20, 10)
  line L851 (30, 10) -> (25.5, 10)
  line L852 (-15, 20) -> (-19.5, 20)
  line L853 (25.5, 24.5) -> (30, 24.5)
  line L854 (30.5, 20) -> (30.5, 24.5)
  line L855 (25, 19.5) -> (25, 15)
  line L856 (-19.5, 20) -> (-19.5, 24.5)
  line L857 (-15, 29.5) -> (-15, 25)
  line L858 (35, 14.5) -> (35, 10)
  line L859 (-29.5, 20) -> (-29.5, 24.5)
  line L860 (-24.5, 25) -> (-24.5, 29.5)
  line L861 (-15, 14.5) -> (-15, 10)
  line L862 (25.5, 15) -> (25.5, 19.5)
  line L863 (30.5, 19.5) -> (35, 19.5)
  line L864 (-15, 19.5) -> (-15, 15)
  line L865 (-34.5, 29.5) -> (-30, 29.5)
  line L866 (-20, 24.5) -> (-20, 20)
  line L867 (25, 20) -> (20.5, 20)
  line L868 (-24.5, 20) -> (-24.5, 24.5)
  line L869 (-20, 10) -> (-24.5, 10)
  line L870 (-15, 24.5) -> (-15, 20)
  line L871 (25.5, 10) -> (25.5, 14.5)
  line L872 (30.5, 15) -> (30.5, 19.5)
  line L873 (-25, 19.5) -> (-25, 15)
  line L874 (-15, 15) -> (-19.5, 15)
  line L875 (35, 15) -> (30.5, 15)
  line L876 (-30, 10) -> (-34.5, 10)
  line L877 (35, 19.5) -> (35, 15)
  line L878 (-14.5, 10) -> (-14.5, 14.5)
  line L879 (20.5, 24.5) -> (25, 24.5)
  line L880 (-20, 15) -> (-24.5, 15)
  line L881 (-30, 25) -> (-34.5, 25)
  line L882 (-15, 10) -> (-19.5, 10)
  line L883 (25.5, 14.5) -> (30, 14.5)
  line L884 (20.5, 29.5) -> (25, 29.5)
  line L885 (5, 15) -> (0.5, 15)
  line L886 (5, 14.5) -> (5, 10)
  line L887 (5, 10) -> (0.5, 10)
  line L888 (0.5, 10) -> (0.5, 14.5)
  line L889 (0.5, 14.5) -> (5, 14.5)
  line L890 (0.5, 19.5) -> (5, 19.5)
  line L891 (5, 24.5) -> (5, 20)
  line L892 (0.5, 25) -> (0.5, 29.5)
  line L893 (5, 20) -> (0.5, 20)
  line L894 (0, 19.5) -> (0, 15)
  line L895 (0.5, 15) -> (0.5, 19.5)
  line L896 (0, 30) -> (-4.5, 30)
  line L897 (-29.5, 34.5) -> (-25, 34.5)
  line L898 (-30, 30) -> (-34.5, 30)
  line L899 (-20, 34.5) -> (-20, 30)
  line L900 (-19.5, 30) -> (-19.5, 34.5)
  line L901 (-24.5, 34.5) -> (-20, 34.5)
  line L902 (-10, 34.5) -> (-10, 30)
  line L903 (-24.5, 30) -> (-24.5, 34.5)
  line L904 (-34.5, 30) -> (-34.5, 34.5)
  line L905 (-9.5, 30) -> (-9.5, 34.5)
  line L906 (-34.5, 34.5) -> (-30, 34.5)
  line L907 (-15, 30) -> (-19.5, 30)
  line L908 (-14.5, 30) -> (-14.5, 34.5)
  line L909 (-14.5, 34.5) -> (-10, 34.5)
  line L910 (-30, 34.5) -> (-30, 30)
  line L911 (-29.5, 30) -> (-29.5, 34.5)
  line L912 (-20, 30) -> (-24.5, 30)
  line L913 (-25, 30) -> (-29.5, 30)
  line L914 (-25, 34.5) -> (-25, 30)
  line L915 (5, 34.5) -> (5, 30)
  line L916 (30, 34.5) -> (30, 30)
  line L917 (-15, 34.5) -> (-15, 30)
  line L918 (-9.5, 34.5) -> (-5, 34.5)
  line L919 (-4.5, 34.5) -> (0, 34.5)
  line L920 (30.5, 30) -> (30.5, 34.5)
  line L921 (-4.5, 30) -> (-4.5, 34.5)
  line L922 (20, 30) -> (15.5, 30)
  line L923 (25.5, 34.5) -> (30, 34.5)
  line L924 (15.5, 34.5) -> (20, 34.5)
  line L925 (-10, 30) -> (-14.5, 30)
  line L926 (-19.5, 34.5) -> (-15, 34.5)
  line L927 (-5, 34.5) -> (-5, 30)
  line L928 (-5, 30) -> (-9.5, 30)
  line L929 (20.5, 34.5) -> (25, 34.5)
  line L930 (35, 34.5) -> (35, 30)
  line L931 (5.5, 34.5) -> (10, 34.5)
  line L932 (15, 30) -> (10.5, 30)
  line L933 (0.5, 30) -> (0.5, 34.5)
  line L934 (10.5, 34.5) -> (15, 34.5)
  line L935 (5, 30) -> (0.5, 30)
  line L936 (10, 30) -> (5.5, 30)
  line L937 (15, 34.5) -> (15, 30)
  line L938 (10, 34.5) -> (10, 30)
  line L939 (5.5, 30) -> (5.5, 34.5)
  line L940 (0.5, 34.5) -> (5, 34.5)
  line L941 (0, 34.5) -> (0, 30)
  line L942 (15.5, 30) -> (15.5, 34.5)
  line L943 (10.5, 30) -> (10.5, 34.5)
  line L944 (30, 30) -> (25.5, 30)
  line L945 (35, 30) -> (30.5, 30)
  line L946 (25, 30) -> (20.5, 30)
  line L947 (25.5, 30) -> (25.5, 34.5)
  line L948 (20, 34.5) -> (20, 30)
  line L949 (20.5, 30) -> (20.5, 34.5)
  line L950 (25, 34.5) -> (25, 30)
  line L951 (30.5, 34.5) -> (35, 34.5)
  line L952 (0, -35) -> (-4.5, -35)
  line L953 (-29.5, -30.5) -> (-25, -30.5)
  line L954 (-30, -35) -> (-34.5, -35)
  line L955 (-20, -30.5) -> (-20, -35)
  line L956 (-19.5, -35) -> (-19.5, -30.5)
  line L957 (-24.5, -30.5) -> (-20, -30.5)
  line L958 (-10, -30.5) -> (-10, -35)
  line L959 (-24.5, -35) -> (-24.5, -30.5)
  line L960 (-34.5, -35) -> (-34.5, -30.5)
  line L961 (-9.5, -35) -> (-9.5, -30.5)
  line L962 (-34.5, -30.5) -> (-30, -30.5)
  line L963 (-15, -35) -> (-19.5, -35)
  line L964 (-14.5, -35) -> (-14.5, -30.5)
  line L965 (-14.5, -30.5) -> (-10, -30.5)
  line L966 (-30, -30.5) -> (-30, -35)
  line L967 (-29.5, -35) -> (-29.5, -30.5)
  line L968 (-20, -35) -> (-24.5, -35)
  line L969 (-25, -35) -> (-29.5, -35)
  line L970 (-25, -30.5) -> (-25, -35)
  line L971 (5, -30.5) -> (5, -35)
  line L972 (30, -30.5) -> (30, -35)
  line L973 (-15, -30.5) -> (-15, -35)
  line L974 (-9.5, -30.5) -> (-5, -30.5)
  line L975 (-4.5, -30.5) -> (0, -30.5)
  line L976 (30.5, -35) -> (30.5, -30.5)
  line L977 (-4.5, -35) -> (-4.5, -30.5)
  line L978 (20, -35) -> (15.5, -35)
  line L979 (25.5, -30.5) -> (30, -30.5)
  line L980 (15.5, -30.5) -> (20, -30.5)
  line L981 (-10, -35) -> (-14.5, -35)
  line L982 (-19.5, -30.5) -> (-15, -30.5)
  line L983 (-5, -30.5) -> (-5, -35)
  line L984 (-5, -35) -> (-9.5, -35)
  line L985 (20.5, -30.5) -> (25, -30.5)
  line L986 (35, -30.5) -> (35, -35)
  line L987 (5.5, -30.5) -> (10, -30.5)
  line L988 (15, -35) -> (10.5, -35)
  line L989 (0.5, -35) -> (0.5, -30.5)
  line L990 (10.5, -30.5) -> (15, -30.5)
  line L991 (5, -35) -> (0.5, -35)
  line L992 (10, -35) -> (5.5, -35)
  line L993 (15, -30.5) -> (15, -35)
  line L994 (10, -30.5) -> (10, -35)
  line L995 (5.5, -35) -> (5.5, -30.5)
  line L996 (0.5, -30.5) -> (5, -30.5)
  line L997 (0, -30.5) -> (0, -35)
  line L998 (15.5, -35) -> (15.5, -30.5)
  line L999 (10.5, -35) -> (10.5, -30.5)
  line L1000 (30, -35) -> (25.5, -35)
  line L1001 (35, -35) -> (30.5, -35)
  line L1002 (25, -35) -> (20.5, -35)
  line L1003 (25.5, -35) -> (25.5, -30.5)
  line L1004 (20, -30.5) -> (20, -35)
  line L1005 (20.5, -35) -> (20.5, -30.5)
  line L1006 (25, -30.5) -> (25, -35)
  line L1007 (30.5, -30.5) -> (35, -30.5)
  line L1008 (39, -40) -> (-36, -40)
  line L1009 (-36, -40) -> (-36, 37)
  line L1010 (-36, 37) -> (39, 37)
  line L1011 (39, 37) -> (39, -40)
  point P0 (-4.5, 29.5)
  point P1 (-9.5, 29.5)
  point P2 (-29.5, 29.5)
  point P3 (-14.5, 29.5)
  point P4 (-34.5, 29.5)
  point P5 (10.5, 29.5)
  point P6 (35, 29.5)
  point P7 (30, 29.5)
  point P8 (-19.5, 29.5)
  point P9 (-24.5, 29.5)
  point P10 (0.5, 29.5)
  point P11 (25, 29.5)
  point P12 (-10, 29.5)
  point P13 (15, 29.5)
  point P14 (5.5, 29.5)
  point P15 (-5, 29.5)
  point P16 (-15, 29.5)
  point P17 (5, 29.5)
  point P18 (20, 29.5)
  point P19 (-20, 29.5)
  point P20 (10, 29.5)
  point P21 (-30, 29.5)
  point P22 (-25, 29.5)
  point P23 (30.5, 29.5)
  point P24 (15.5, 29.5)
  point P25 (0, 29.5)
  point P26 (20.5, 29.5)
  point P27 (25.5, 29.5)
  point P28 (-4.5, -35.5)
  point P29 (-9.5, -35.5)
  point P30 (-29.5, -35.5)
  point P31 (-14.5, -35.5)
  point P32 (-34.5, -35.5)
  point P33 (10.5, -35.5)
  point P34 (35, -35.5)
  point P35 (30, -35.5)
  point P36 (-19.5, -35.5)
  point P37 (-24.5, -35.5)
  point P38 (0.5, -35.5)
  point P39 (25, -35.5)
  point P40 (-10, -35.5)
  point P41 (15, -35.5)
  point P42 (5.5, -35.5)
  point P43 (-5, -35.5)
  point P44 (-15, -35.5)
  point P45 (5, -35.5)
  point P46 (20, -35.5)
  point P47 (-20, -35.5)
  point P48 (10, -35.5)
  point P49 (-30, -35.5)
  point P50 (-25, -35.5)
  point P51 (30.5, -35.5)
  point P52 (15.5, -35.5)
  point P53 (0, -35.5)
  point P54 (20.5, -35.5)
  point P55 (25.5, -35.5)
  dimension "d10" = 4.5
  dimension "d11" = 4.5
  dimension "d12" = 4.5
  dimension "d13" = 4.5
  dimension "d14" = 4.5
  dimension "d15" = 4.5
  dimension "d16" = 4.5
  dimension "d17" = 4.5
  dimension "d18" = 4.5
  dimension "d19" = 4.5
  dimension "d20" = 4.5
  dimension "d21" = 4.5
  dimension "d22" = 4.5
  dimension "d23" = 4.5
  dimension "d24" = 4.5
  dimension "d25" = 4.5
  dimension "d26" = 4.5
  dimension "d27" = 4.5
  dimension "d28" = 4.5
  dimension "d29" = 4.5
  dimension "d30" = 4.5
  dimension "d31" = 4.5
  dimension "d32" = 4.5
  dimension "d33" = 4.5
  dimension "d34" = 4.5
  dimension "d35" = 4.5
  dimension "d36" = 4.5
  dimension "d37" = 4.5
  dimension "d38" = 4.5
  dimension "d39" = 4.5
  dimension "d40" = 4.5
  dimension "d41" = 4.5
  dimension "d42" = 4.5
  dimension "d43" = 4.5
  dimension "d44" = 4.5
  dimension "d45" = 4.5
  dimension "d46" = 4.5
  dimension "d47" = 4.5
  dimension "d48" = 4.5
  dimension "d49" = 4.5
  dimension "d50" = 4.5
  dimension "d51" = 4.5
  dimension "d52" = 4.5
  dimension "d53" = 4.5
  dimension "d54" = 4.5
  dimension "d55" = 4.5
  dimension "d56" = 4.5
  dimension "d57" = 4.5
  dimension "d58" = 4.5
  dimension "d59" = 4.5
  dimension "d60" = 4.5
  dimension "d61" = 4.5
  dimension "d62" = 4.5
  dimension "d63" = 4.5
  dimension "d64" = 4.5
  dimension "d65" = 4.5
  dimension "d66" = 4.5
  dimension "d67" = 4.5
  dimension "d68" = 4.5
  dimension "d69" = 4.5
  dimension "d70" = 4.5
  dimension "d71" = 4.5
  dimension "d72" = 4.5
  dimension "d73" = 4.5
  dimension "d74" = 4.5
  dimension "d75" = 4.5
  dimension "d76" = 4.5
  dimension "d77" = 4.5
  dimension "d78" = 4.5
  dimension "d79" = 4.5
  dimension "d80" = 4.5
  dimension "d81" = 4.5
  dimension "d82" = 4.5
  dimension "d83" = 4.5
  dimension "d84" = 4.5
  dimension "d85" = 4.5
  dimension "d86" = 4.5
  dimension "d87" = 4.5
  dimension "d88" = 4.5
  dimension "d89" = 4.5
  dimension "d90" = 4.5
  dimension "d91" = 4.5
  dimension "d92" = 4.5
  dimension "d93" = 4.5
  dimension "d94" = 4.5
  dimension "d95" = 4.5
  dimension "d96" = 4.5
  dimension "d97" = 4.5
  dimension "d98" = 4.5
  dimension "d99" = 4.5
  dimension "d100" = 4.5
  dimension "d101" = 4.5
  dimension "d102" = 4.5
  dimension "d103" = 4.5
  dimension "d104" = 4.5
  dimension "d105" = 4.5
  dimension "d106" = 4.5
  dimension "d107" = 4.5
  dimension "d108" = 4.5
  dimension "d109" = 4.5
  dimension "d110" = 4.5
  dimension "d111" = 4.5
  dimension "d112" = 4.5
  dimension "d113" = 4.5
  dimension "d114" = 4.5
  dimension "d115" = 4.5
  dimension "d116" = 4.5
  dimension "d117" = 4.5
  dimension "d118" = 4.5
  dimension "d119" = 4.5
  dimension "d120" = 4.5
  dimension "d121" = 4.5
  dimension "d122" = 4.5
  dimension "d123" = 4.5
  dimension "d124" = 4.5
  dimension "d125" = 4.5
  dimension "d126" = 4.5
  dimension "d127" = 4.5
  dimension "d128" = 4.5
  dimension "d129" = 4.5
  dimension "d130" = 4.5
  dimension "d131" = 4.5
  dimension "d132" = 4.5
  dimension "d133" = 4.5
  dimension "d134" = 4.5
  dimension "d135" = 4.5
  dimension "d136" = 4.5
  dimension "d137" = 4.5
  dimension "d138" = 4.5
  dimension "d139" = 4.5
  dimension "d140" = 4.5
  dimension "d141" = 4.5
  dimension "d142" = 4.5
  dimension "d143" = 4.5
  dimension "d144" = 4.5
  dimension "d145" = 4.5
  dimension "d146" = 4.5
  dimension "d147" = 4.5
  dimension "d148" = 4.5
  dimension "d149" = 4.5
  dimension "d150" = 4.5
  dimension "d151" = 4.5
  dimension "d152" = 4.5
  dimension "d153" = 4.5
  dimension "d154" = 4.5
  dimension "d155" = 4.5
  dimension "d156" = 4.5
  dimension "d157" = 4.5
  dimension "d158" = 4.5
  dimension "d159" = 4.5
  dimension "d160" = 4.5
  dimension "d161" = 4.5
  dimension "d162" = 4.5
  dimension "d163" = 4.5
  dimension "d164" = 4.5
  dimension "d165" = 4.5
  dimension "d166" = 4.5
  dimension "d167" = 4.5
  dimension "d168" = 4.5
  dimension "d169" = 4.5
  dimension "d170" = 4.5
  dimension "d171" = 4.5
  dimension "d172" = 4.5
  dimension "d173" = 4.5
  dimension "d174" = 4.5
  dimension "d175" = 4.5
  dimension "d176" = 4.5
  dimension "d177" = 4.5
  dimension "d178" = 4.5
  dimension "d179" = 4.5
  dimension "d180" = 4.5
  dimension "d181" = 4.5
  dimension "d182" = 4.5
  dimension "d183" = 4.5
  dimension "d184" = 4.5
  dimension "d185" = 4.5
  dimension "d186" = 4.5
  dimension "d187" = 4.5
  dimension "d188" = 4.5
  dimension "d189" = 4.5
  dimension "d190" = 4.5
  dimension "d191" = 4.5
  dimension "d192" = 4.5
  dimension "d193" = 4.5
  dimension "d194" = 4.5
  dimension "d195" = 4.5
  dimension "d196" = 4.5
  dimension "d197" = 4.5
  dimension "d198" = 4.5
  dimension "d199" = 4.5
  dimension "d200" = 4.5
  dimension "d201" = 4.5
  dimension "d202" = 4.5
  dimension "d203" = 4.5
  dimension "d204" = 4.5
  dimension "d205" = 4.5
  dimension "d206" = 4.5
  dimension "d207" = 4.5
  dimension "d208" = 4.5
  dimension "d209" = 4.5
  dimension "d210" = 4.5
  dimension "d211" = 4.5
  dimension "d212" = 4.5
  dimension "d213" = 4.5
  dimension "d214" = 4.5
  dimension "d215" = 4.5
  dimension "d216" = 4.5
  dimension "d217" = 4.5
  dimension "d218" = 4.5
  dimension "d219" = 4.5
  dimension "d220" = 4.5
  dimension "d221" = 4.5
  dimension "d222" = 4.5
  dimension "d223" = 4.5
  dimension "d224" = 4.5
  dimension "d225" = 4.5
  dimension "d226" = 4.5
  dimension "d227" = 4.5
  dimension "d228" = 4.5
  dimension "d229" = 4.5
  dimension "d230" = 4.5
  dimension "d231" = 4.5
  dimension "d232" = 4.5
  dimension "d233" = 4.5
  dimension "d234" = 4.5
  dimension "d235" = 4.5
  dimension "d236" = 4.5
  dimension "d237" = 4.5
  dimension "d238" = 4.5
  dimension "d239" = 4.5
  dimension "d240" = 4.5
  dimension "d241" = 4.5
  dimension "d242" = 4.5
  dimension "d243" = 4.5
  dimension "d244" = 4.5
  dimension "d245" = 4.5
  dimension "d246" = 4.5
  dimension "d247" = 4.5
  dimension "d248" = 4.5
  dimension "d249" = 4.5
  dimension "d250" = 4.5
  dimension "d251" = 4.5
  dimension "d252" = 4.5
  dimension "d253" = 4.5
  dimension "d254" = 4.5
  dimension "d255" = 4.5
  dimension "d256" = 4.5
  dimension "d257" = 4.5
  dimension "d258" = 4.5
  dimension "d259" = 4.5
  dimension "d260" = 4.5
  dimension "d261" = 4.5
  dimension "d262" = 4.5
  dimension "d263" = 4.5
  dimension "d264" = 4.5
  dimension "d265" = 4.5
  dimension "d266" = 4.5
  dimension "d267" = 4.5
  dimension "d268" = 4.5
  dimension "d269" = 4.5
  dimension "d270" = 4.5
  dimension "d271" = 4.5
  dimension "d272" = 4.5
  dimension "d273" = 4.5
  dimension "d274" = 4.5
  dimension "d275" = 4.5
  dimension "d276" = 4.5
  dimension "d277" = 4.5
  dimension "d278" = 4.5
  dimension "d279" = 4.5
  dimension "d280" = 4.5
  dimension "d281" = 4.5
  dimension "d282" = 4.5
  dimension "d283" = 4.5
  dimension "d284" = 4.5
  dimension "d285" = 4.5
  dimension "d286" = 4.5
  dimension "d287" = 4.5
  dimension "d288" = 4.5
  dimension "d289" = 4.5
  dimension "d290" = 4.5
  dimension "d291" = 4.5
  dimension "d292" = 4.5
  dimension "d293" = 4.5
  dimension "d294" = 4.5
  dimension "d295" = 4.5
  dimension "d296" = 4.5
  dimension "d297" = 4.5
  dimension "d298" = 4.5
  dimension "d299" = 4.5
  dimension "d300" = 4.5
  dimension "d301" = 4.5
  dimension "d302" = 4.5
  dimension "d303" = 4.5
  dimension "d304" = 4.5
  dimension "d305" = 4.5
  dimension "d306" = 4.5
  dimension "d307" = 4.5
  dimension "d308" = 4.5
  dimension "d309" = 4.5
  dimension "d310" = 4.5
  dimension "d311" = 4.5
  dimension "d312" = 4.5
  dimension "d313" = 4.5
  dimension "d314" = 4.5
  dimension "d315" = 4.5
  dimension "d316" = 4.5
  dimension "d317" = 4.5
  dimension "d318" = 4.5
  dimension "d319" = 4.5
  dimension "d320" = 4.5
  dimension "d321" = 4.5
  dimension "d322" = 4.5
  dimension "d323" = 4.5
  dimension "d324" = 4.5
  dimension "d325" = 4.5
  dimension "d326" = 4.5
  dimension "d327" = 4.5
  dimension "d328" = 4.5
  dimension "d329" = 4.5
  dimension "d330" = 4.5
  dimension "d331" = 4.5
  dimension "d332" = 4.5
  dimension "d333" = 4.5
  dimension "d334" = 4.5
  dimension "d335" = 4.5
  dimension "d336" = 4.5
  dimension "d337" = 4.5
  dimension "d338" = 4.5
  dimension "d339" = 4.5
  dimension "d340" = 4.5
  dimension "d341" = 4.5
  dimension "d342" = 4.5
  dimension "d343" = 4.5
  dimension "d344" = 4.5
  dimension "d345" = 4.5
  dimension "d346" = 4.5